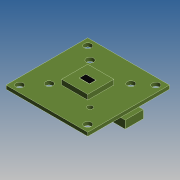
# Autodesk Inventor part: F103
Saved by Autodesk Inventor 2019 (Build 230136000, 136)
## iProperties
Created: 2015-02-04
Part Number: F103
Material: Acetal Resin, Black
Document SubType Name: Modeling
Designer: serge.amoos
Density: 1.425 g/cm^3
Appearance: Olive Green
Description: Caméra USB
Author: serge.amoos
Autodesk Inventor part; units mm, degrees
ref_plane "YZ Plane" through (0, 0, 0) normal (1, 0, 0) x (0, 1, 0)
ref_plane "XZ Plane" through (0, 0, 0) normal (0, 1, 0) x (-1, 0, 0)
ref_plane "XY Plane" through (0, 0, 0) normal (0, 0, 1) x (1, 0, 0)
sketch "Sketch1" plane through (0, 0, 0) normal (0, 0, 1) x (1, 0, 0)
  line L0 (-25.2, 0) -> (25.2, 0) construction
  line L1 (0, -25.2) -> (0, 25.2) construction
  line L2 (-18, 18) -> (18, 18)
  line L3 (18, 18) -> (18, -18)
  line L4 (18, -18) -> (-18, -18)
  line L5 (-18, -18) -> (-18, 18)
  point P0 (0, 0)
  point P1 (0, 18)
  point P2 (18, 0)
  dimension "d0" = 36
  dimension "d1" = 36
  constraints: 8 end point, 2 midpoint, 2 parallel, 2 point on line, 1 horizontal, 1 perpendicular
  measures "d0" distance of L2.start L2.end
  measures "d1" distance of L2.end L3.end
extrude "Extrusion1" add sketch "Sketch1" along normal blind 1.6
sketch "Sketch2" plane through (0, 0, 1.6) normal (0, 0, 1) x (1, 0, 0)
  point P0 (0, 0)
  point P1 (-15, 15)
  dimension "d4" = 15
  dimension "d5" = 15
  measures "d4" horizontal distance of point (-15, 15) point (0, 0)
  measures "d5" horizontal distance of point (0, 0) point (-15, 15)
hole "Hole1" at (-15, 15, 1.6) direction (0, 0, -1) diameter 3.2 end through all
pattern_circular "Circular Pattern1" count 4 over 360 about axis through (0, 0, -10) along (0, 0, 1) of "Hole1"
sketch "Sketch3" plane through (0, 0, 1.6) normal (0, 0, 1) x (1, 0, 0)
  line L0 (-25.2, 0) -> (25.2, 0) construction
  line L1 (0, -25.2) -> (0, 25.2) construction
  line L2 (-2.256, 1.44) -> (2.256, 1.44)
  line L3 (2.256, 1.44) -> (2.256, -1.44)
  line L4 (2.256, -1.44) -> (-2.256, -1.44)
  line L5 (-2.256, -1.44) -> (-2.256, 1.44)
  point P0 (0, 0)
  point P1 (0, 1.44)
  point P2 (2.256, 0)
  dimension "d16" = 4.512
  dimension "d17" = 2.88
  constraints: 8 end point, 2 midpoint, 2 parallel, 2 point on line, 1 horizontal, 1 perpendicular
  measures "d16" distance of L2.start L2.end
  measures "d17" distance of L2.end L3.end
extrude "Extrusion2" add sketch "Sketch3" along normal blind 2.3
sketch "Sketch4" plane through (0, 0, 1.6) normal (0, 0, 1) x (1, 0, 0)
  line L0 (-5.75, 5.75) -> (5.75, 5.75)
  line L1 (5.75, 5.75) -> (5.75, -5.75)
  line L2 (5.75, -5.75) -> (-5.75, -5.75)
  line L3 (-5.75, -5.75) -> (-5.75, 5.75)
  line L4 (-25.2, 0) -> (25.2, 0) construction
  line L5 (0, -25.2) -> (0, 25.2) construction
  point P0 (0, 0)
  point P1 (0, 5.75)
  point P2 (5.75, 0)
  dimension "d20" = 11.5
  dimension "d21" = 11.5
  constraints: 8 end point, 2 midpoint, 2 parallel, 2 point on line, 1 horizontal, 1 perpendicular
  measures "d20" distance of L0.start L0.end
  measures "d21" distance of L0.end L1.end
extrude "Extrusion3" add sketch "Sketch4" along normal blind 2.2
sketch "Sketch5" plane through (0, 0, 1.6) normal (0, 0, 1) x (1, 0, 0)
  point P0 (0, 0)
sketch "Sketch6" plane through (0, 0, 0) normal (0, 0, -1) x (-1, 0, 0)
  line L0 (25.2, 0) -> (-25.2, 0) projected
  line L1 (0, -25.2) -> (0, 25.2) projected
  line L2 (-20, 4.5) -> (-11, 4.5)
  line L3 (-11, 4.5) -> (-11, -3.5)
  line L4 (-11, -3.5) -> (-20, -3.5)
  line L5 (-20, -3.5) -> (-20, 4.5)
  line L6 (-18, 18) -> (-18, -18) projected
  line L7 (-18, -18) -> (18, -18) projected
  point P0 (0, 0)
  point P1 (-11, 0.5)
  dimension "d24" = 9
  dimension "d25" = 8
  dimension "d26" = 2
  dimension "d58" = 18.5
  constraints: 8 end point, 2 parallel, 1 horizontal, 1 midpoint, 1 perpendicular
  measures "d24" distance of L2.start L2.end
  measures "d25" distance of L4.end L2.start
  measures "d26" distance between parallel lines of L6 L5
  measures "d58" distance from line of L7 point (-11, 0.5)
extrude "Extrusion4" add sketch "Sketch6" along normal blind 3.5 contours L3 L4 L6 L0 | L0 L6 L2 L3 | L6 L4 L5 L0 | L0 L5 L2 L6
sketch "Sketch7" plane through (0, 0, 1.6) normal (0, 0, 1) x (1, 0, 0)
  line L0 (-25.6, 0) -> (27.6, 0) projected
  line L1 (0, -25.2) -> (0, 25.2) projected
  line L2 (18, -18) -> (18, 18) projected
  line L3 (18, -18) -> (-18, -18) projected
  circle A0 centre (9, -8) radius 1.15
  circle A1 centre (-9, -8) radius 1.6
  circle A2 centre (-9, 10) radius 1.6
  circle A3 centre (9, 10) radius 1.6
  line L4 (-18, 18) -> (18, 18) projected
  point P0 (0, 0)
  dimension "d44" = 3.2
  dimension "d45" = 3.2
  dimension "d46" = 3.2
  dimension "d47" = 2.3
  dimension "d48" = 10
  dimension "d49" = 10
  dimension "d50" = 9
  dimension "d51" = 9
  dimension "d52" = 8
  dimension "d53" = 8
  dimension "d54" = 18
  dimension "d55" = 18
  constraints: 4 centre point
  measures "d44" diameter of A1
  measures "d45" diameter of A2
  measures "d46" diameter of A3
  measures "d47" diameter of A0
  measures "d48" distance from line of L3 A1.centre
  measures "d49" distance from line of L3 A0.centre
  measures "d50" distance from line of L2 A0.centre
  measures "d51" distance from line of L2 A3.centre
  measures "d52" distance from line of L4 A3.centre
  measures "d53" distance from line of L4 A2.centre
  measures "d54" distance of A3.centre A2.centre
  measures "d55" distance of A0.centre A1.centre
extrude "Extrusion5" cut sketch "Sketch7" against normal through all contours A0 | A1 | A2 | A3
equation "\"d20\" = d21"
body "Solid1"
